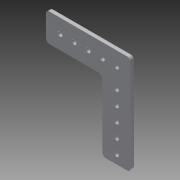
# Autodesk Inventor part: Roller Crossbar Gusset (Custom)
Saved by Autodesk Inventor 2014 (Build 180170000, 170)
## iProperties
Created: 2014-01-20
Part Number: Roller Crossbar Gusset (Custom)
Material: Aluminum 6061
Document SubType Name: Modeling
Designer: Michael
Density: 2.71 g/cm^3
Appearance: Aluminum - Flat
Author: Michael
Autodesk Inventor part; units mm, degrees
ref_plane "YZ Plane" through (0, 0, 0) normal (1, 0, 0) x (0, 1, 0)
ref_plane "XZ Plane" through (0, 0, 0) normal (0, 1, 0) x (-1, 0, 0)
ref_plane "XY Plane" through (0, 0, 0) normal (0, 0, 1) x (1, 0, 0)
sketch "Sketch1" plane through (0, 0, 0) normal (0, 0, 1) x (1, 0, 0)
  line L0 (0, 0) -> (76.2, 0)
  line L1 (76.2, 0) -> (76.2, -88.9)
  line L2 (76.2, -88.9) -> (50.8, -88.9)
  line L3 (50.8, -88.9) -> (50.8, -25.4)
  line L4 (50.8, -25.4) -> (0, -25.4)
  line L5 (0, -25.4) -> (0, 0)
  circle A0 centre (12.7, -12.7) radius 2.0701
  circle A1 centre (63.5, -30.1625) radius 2.0701
  circle A2 centre (63.5, -42.8625) radius 2.0701
  circle A3 centre (63.5, -55.5625) radius 2.0701
  circle A4 centre (63.5, -68.2625) radius 2.0701
  circle A5 centre (63.5, -80.9625) radius 2.0701
  circle A6 centre (25.4, -12.7) radius 2.0701
  circle A7 centre (38.1, -12.7) radius 2.0701
  circle A8 centre (50.8, -12.7) radius 2.0701
  circle A9 centre (63.5, -12.7) radius 2.0701
  dimension "d0" = 76.2
  dimension "d3" = 25.4
  dimension "d4" = 88.9
  dimension "d5" = 4.1402
  dimension "d6" = 12.7
  dimension "d7" = 12.7
  dimension "d18" = 12.7
  dimension "d23" = 12.7
  dimension "d27" = 4.7625
  dimension "d28" = 25.4
  dimension "d31" = 12.7
  constraints: 12 end point, 10 centre point, 4 vertical, 2 horizontal, 2 parallel, 1 equal radius, 16 other
  measures "d0" distance of L0.end L0.start
  measures "d3" distance of L1.end L2.end
  measures "d4" distance between parallel lines of L0 L2
  measures "d5" diameter of A0
  measures "d6" distance from line of L4 A0.centre
  measures "d7" distance from line of L5 A0.centre
  measures "d18" distance of A1.centre A2.centre
  measures "d23" distance from line of L3 A1.centre
  measures "d27" distance from line of L4 A1.centre
  measures "d28" distance of L4.end L0.start
  measures "d31" distance of A0.centre A6.centre
extrude "Extrusion1" add sketch "Sketch1" along normal blind 3.175
fillet "Fillet1" radius 3.175 6 edges at (0, 0, 1.5875) (0, -25.4, 1.5875) (50.8, -25.4, 1.5875) (50.8, -88.9, 1.5875) (76.2, -88.9, 1.5875) (76.2, 0, 1.5875)
body "Solid1"
